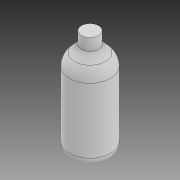
# Autodesk Inventor part: 2L bottle
Saved by Autodesk Inventor 2020 (Build 240168000, 168)
## iProperties
Created: 2021-05-05
Part Number: 2L bottle
Material: Generic
Document SubType Name: Modeling
Designer: DDeGo
Density: 1 g/cm^3
Appearance: Default
Author: DDeGo
Autodesk Inventor part; units mm, degrees
ref_plane "YZ Plane" through (0, 0, 0) normal (1, 0, 0) x (0, 1, 0)
ref_plane "XZ Plane" through (0, 0, 0) normal (0, 1, 0) x (-1, 0, 0)
ref_plane "XY Plane" through (0, 0, 0) normal (0, 0, 1) x (1, 0, 0)
sketch "Sketch1" plane through (0, 0, 0) normal (0, 0, 1) x (1, 0, 0)
  line L0 (0, 0) -> (40, 0)
  line L1 (60, 20) -> (60, 209.2893)
  line L2 (45.3553, 244.6447) -> (25, 265)
  line L3 (25, 265) -> (25, 300)
  line L4 (25, 300) -> (0, 300)
  line L5 (0, 300) -> (0, 0)
  arc A0 (60, 209.2893) -> (45.3553, 244.6447) centre (10, 209.2893) ccw
  arc A1 (40, 0) -> (60, 20) centre (40, 20) ccw
  point P0 (60, 0)
  dimension "d0" = 300
  dimension "d1" = 60
  dimension "d2" = 135
  dimension "d3" = 35
  dimension "d4" = 50
  dimension "d6" = 25
  dimension "d7" = 20
  constraints: 12 end point, 4 point on circle, 4 tangent, 3 perpendicular, 2 centre point, 2 point on line, 1 horizontal, 1 parallel
  measures "d0" distance between parallel lines of L4 L0
  measures "d1" distance between parallel lines of L1 L5
  measures "d2" angle of L1 L2
  measures "d3" distance of L2.end L3.end
  measures "d4" radius of A0
  measures "d6" distance between parallel lines of L5 L3
  measures "d7" radius of A1
revolve "Revolution1" add sketch "Sketch1" angle 360 about axis through (0, 300, 0) along (0, -1, 0)
body "Solid1"
